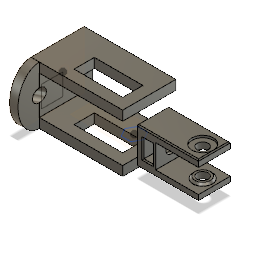
_Y Tensioner.c738b04c-2ad9-4713-af64-9a0c1ec9e032 (Autodesk Fusion 360 design; units mm, degrees)
Autodesk Fusion 360 part; units mm, degrees
sketch "Sketch1" plane through (0, 0, 0) normal (0, 0, 1) x (1, 0, 0)
  line L0 (0, 0) -> (29, 0)
  line L1 (29, 0) -> (29, 17)
  line L2 (29, 17) -> (0, 17)
  line L3 (0, 17) -> (0, 0)
  line L4 (8.977, 3) -> (29.9497, 3)
  line L5 (29.9497, 3) -> (29.9497, 14)
  line L6 (29.9497, 14) -> (8.977, 14)
  line L7 (8.977, 14) -> (8.977, 3)
  dimension "d1" = 17
  dimension "d2" = 29
  measures "d1" distance of L0.start
  measures "d2" distance of L0.start
extrude "Extrude1" add sketch "Sketch1" along normal blind 15 contours L0 L1 L2 L3 L4 L6 L7 makes body 1
sketch "Sketch2" plane through (0, 0, 0) normal (-1, 0, 0) x (0, 0, 1)
  line L0 (0, 17) -> (0, 0)
  line L1 (0, 0) -> (15, 0)
  line L2 (15, 0) -> (15, 17)
  line L3 (15, 17) -> (0, 17)
  circle A0 centre (7.5, 8.5) radius 3.1
  dimension "d5" = 6.2
  measures "d5" diameter of A0
extrude "Extrude2" cut sketch "Sketch2" against normal blind 3 draft -10 contours A0 bodies 1
sketch "Sketch3" plane through (0, 0, 0) normal (0, -1, 0) x (1, 0, 0)
  line L0 (0, 0) -> (29, 0)
  line L1 (29, 0) -> (29, 15)
  line L2 (29, 15) -> (0, 15)
  line L3 (0, 15) -> (0, 0)
  circle A0 centre (23.4671, 7.5) radius 2.6
  dimension "d8" = 5.2
  measures "d8" diameter of A0
extrude "Extrude3" cut sketch "Sketch3" against normal blind 17 contours A0 bodies 1
sketch "Sketch4" plane through (0, 14, 0) normal (0, -1, 0) x (1, 0, 0)
  circle A0 centre (23.4671, 7.5) radius 2.6
  line L0 (8.977, 0) -> (29, 0)
  line L1 (29, 0) -> (29, 15)
  line L2 (29, 15) -> (8.977, 15)
  line L3 (8.977, 15) -> (8.977, 0)
  circle A1 centre (23.4671, 7.5) radius 4.5
  dimension "d11" = 9
  measures "d11" diameter of A1
extrude "Extrude4" add sketch "Sketch4" along normal blind 1 contours A1 bodies 1
chamfer "Chamfer1" distance 0.9 angle 45 1 edges at (19.2716, 13, 5.8727) on bodies 1
sketch "Sketch5" plane through (0, 3, 0) normal (0, 1, 0) x (-1, 0, 0)
  circle A0 centre (-23.4671, 7.5) radius 2.6
  line L0 (-29, 0) -> (-8.977, 0)
  line L1 (-8.977, 0) -> (-8.977, 15)
  line L2 (-8.977, 15) -> (-29, 15)
  line L3 (-29, 15) -> (-29, 0)
  circle A1 centre (-23.4671, 7.5) radius 4.5
  dimension "d15" = 9
  measures "d15" diameter of A1
extrude "Extrude5" add sketch "Sketch5" along normal blind 1 contours A1 bodies 1
chamfer "Chamfer2" distance 0.9 angle 45 1 edges at (27.6626, 4, 5.8727) on bodies 1
sketch "Sketch6" plane through (8.977, 0, 0) normal (1, 0, 0) x (0, 0, -1)
  line L0 (0, 3) -> (0, 14)
  line L1 (0, 14) -> (-15, 14)
  line L2 (-15, 14) -> (-15, 3)
  line L3 (-15, 3) -> (0, 3)
  line L4 (-11.75, 4.25) -> (-3.25, 4.25)
  line L5 (-3.25, 12.75) -> (-11.75, 12.75)
  line L6 (-11.75, 4.25) -> (-3.25, 12.75) construction
  line L7 (-3.25, 4.25) -> (-11.75, 12.75) construction
  line L8 (-5.0463, 12.75) -> (-9.9537, 12.75)
  line L9 (-9.9537, 4.25) -> (-5.0463, 4.25)
  line L10 (-9.9537, 12.75) -> (-16, 12.75)
  line L11 (-16, 12.75) -> (-16, 4.25)
  line L12 (-16, 4.25) -> (-11.75, 4.25)
  line L13 (-2.5925, 8.5) -> (-3.25, 9.6388)
  line L14 (-3.25, 4.25) -> (-3.25, 7.3612)
  line L15 (-3.25, 9.6388) -> (-3.25, 12.75)
  line L16 (-3.25, 7.3612) -> (-2.5925, 8.5)
  dimension "d19" = 8.5
  dimension "d20" = 8.5
extrude "Extrude6" cut sketch "Sketch6" against normal blind 6 contours L2 L4 L5 L8 L9 L10 L12 L13 L14 L15 L16 bodies 1
sketch "Sketch13" plane through (8.977, 0, 0) normal (1, 0, 0) x (0, 0, -1)
  line L0 (-3.25, 4.25) -> (-15, 4.25)
  line L1 (-15, 4.25) -> (-15, 3)
  line L2 (-15, 3) -> (0, 3)
  line L3 (0, 3) -> (0, 14)
  line L4 (0, 14) -> (-15, 14)
  line L5 (-15, 14) -> (-15, 12.75)
  line L6 (-15, 12.75) -> (-3.25, 12.75)
  line L7 (-3.25, 12.75) -> (-3.25, 9.6388)
  line L8 (-3.25, 9.6388) -> (-2.5925, 8.5)
  line L9 (-2.5925, 8.5) -> (-3.25, 7.3612)
  line L10 (-3.25, 7.3612) -> (-3.25, 4.25)
  line L11 (0, 14) -> (-15, 14)
  line L12 (-15, 14) -> (-15, 3)
  line L13 (-15, 3) -> (0, 3)
  line L14 (0, 3) -> (0, 14)
extrude "Extrude13" add sketch "Sketch13" against normal blind 1.5 contours L0 L6 L7 L8 L9 L10 L12 bodies 1
chamfer "Chamfer6" distance 0.5 angle 45 14 edges at (14.5, 0, 15) (0, 0, 7.5) (14.5, 0, 0) (29, 0, 7.5) (0, 8.5, 15) (0, 8.5, 0) (0, 17, 7.5) (2.977, 8.5, 15) (5.227, 12.75, 15) (7.477, 8.5, 15) (5.227, 4.25, 15) (14.5, 17, 0) (29, 17, 7.5) (14.5, 17, 15) on bodies 1
sketch "Sketch14" plane through (8.977, 0, 0) normal (1, 0, 0) x (0, 0, -1)
  line L0 (-15, 14) -> (-15, 3)
  line L1 (-15, 3) -> (0, 3)
  line L2 (0, 3) -> (0, 14)
  line L3 (0, 14) -> (-15, 14)
  circle A0 centre (-7.5, 8.5775) radius 2.75
  dimension "d54" = 5.5
  measures "d54" diameter of A0
extrude "Extrude14" cut sketch "Sketch14" against normal blind 2 contours A0 bodies 1
sketch "Sketch15" plane through (0, 17, 0) normal (0, 1, 0) x (-1, 0, 0)
  circle A0 centre (-23.4671, 7.5) radius 2.6
  line L0 (-28.5, 0.5) -> (-0.5, 0.5)
  line L1 (-0.5, 0.5) -> (-0.5, 14.5)
  line L2 (-0.5, 14.5) -> (-28.5, 14.5)
  line L3 (-28.5, 14.5) -> (-28.5, 0.5)
  circle A1 centre (-23.4671, 7.5) radius 5
  dimension "d57" = 10
  measures "d57" diameter of A1
extrude "Extrude15" cut sketch "Sketch15" against normal blind 1 contours A1 bodies 1
sketch "Sketch16" plane through (0, 0, 0) normal (0, -1, 0) x (1, 0, 0)
  circle A0 centre (23.4671, 7.5) radius 2.6
  line L0 (0.5, 0.5) -> (28.5, 0.5)
  line L1 (28.5, 0.5) -> (28.5, 14.5)
  line L2 (28.5, 14.5) -> (0.5, 14.5)
  line L3 (0.5, 14.5) -> (0.5, 0.5)
  line L4 (18.9671, 7.5) -> (21.2171, 3.6029)
  line L5 (21.2171, 3.6029) -> (25.7171, 3.6029)
  line L6 (25.7171, 3.6029) -> (27.9671, 7.5)
  line L7 (27.9671, 7.5) -> (25.7171, 11.3971)
  line L8 (25.7171, 11.3971) -> (21.2171, 11.3971)
  line L9 (21.2171, 11.3971) -> (18.9671, 7.5)
  dimension "d63" = 4.5
extrude "Extrude17" cut sketch "Sketch16" against normal blind 1 contours L4 L5 L6 L7 L8 L9 bodies 1
extrude "Extrude16" cut sketch "Sketch16" against normal blind 1 contours L4 L5 L6 L7 L8 L9 bodies 1
sketch "Sketch7" plane through (0, 0, 0) normal (0, 0, 1) x (1, 0, 0)
  line L0 (33, 22) -> (-10, 22)
  line L1 (-10, 22) -> (-10, -5)
  line L2 (-10, -5) -> (33, -5)
  line L3 (33, -5) -> (33, 22)
  line L4 (-6.0376, -0.5) -> (33.9624, -0.5)
  line L5 (33.9624, -0.5) -> (33.9624, 17.5)
  line L6 (33.9624, 17.5) -> (-6.0376, 17.5)
  line L7 (-6.0376, 17.5) -> (-6.0376, -0.5)
  line L8 (-6.0376, -0.5) -> (33.9624, 17.5) construction
  line L9 (33.9624, -0.5) -> (-6.0376, 17.5) construction
  dimension "d23" = 18
  dimension "d24" = 40
  measures "d23" distance of origin
extrude "Extrude7" add sketch "Sketch7" along normal blind 25 separate body contours L0 L1 L2 L3 L4 L6 L7 makes body 2
move_body "Move1" bodies 2 to x (1, 0, 0) y (0, 1, 0) z (0, 0, 1) at (0, 0, -2.5)
sketch "Sketch8" plane through (-10, 0, 0) normal (-1, 0, 0) x (0, 0, 1)
  line L0 (-2.5, 22) -> (-2.5, -5)
  line L1 (-2.5, -5) -> (22.5, -5)
  line L2 (22.5, -5) -> (22.5, 22)
  line L3 (22.5, 22) -> (-2.5, 22)
  circle A0 centre (7.5, 8.4834) radius 2.65
  dimension "d27" = 5.3
  measures "d27" diameter of A0
extrude "Extrude8" cut sketch "Sketch8" against normal blind 4 contours A0 bodies 2
move_body "Move2" bodies 1 to x (1, 0, 0) y (0, 1, 0) z (0, 0, 1) at (0, 0, 5)
sketch "Sketch9" plane through (0, 22, 0) normal (0, 1, 0) x (-1, 0, 0)
  line L0 (-33, -2.5) -> (10, -2.5)
  line L1 (10, -2.5) -> (10, 22.5)
  line L2 (10, 22.5) -> (-33, 22.5)
  line L3 (-33, 22.5) -> (-33, -2.5)
  line L4 (-33, 22.5) -> (-22.9998, 12.5)
  line L5 (-18.2498, 17.25) -> (-27.7498, 17.25)
  line L6 (-27.7498, 17.25) -> (-27.7498, 7.75)
  line L7 (-27.7498, 7.75) -> (-18.2498, 7.75)
  line L8 (-18.2498, 7.75) -> (-18.2498, 17.25)
  line L9 (-18.2498, 17.25) -> (-27.7498, 7.75) construction
  line L10 (-27.7498, 17.25) -> (-18.2498, 7.75) construction
  line L11 (-18.2498, 7.75) -> (-5, 7.75)
  line L12 (-5, 7.75) -> (-5, 17.25)
  line L13 (-5, 17.25) -> (-18.2498, 17.25)
  dimension "d31" = 9.5
  dimension "d32" = 9.5
move_body "Move3" bodies 1 to x (1, 0, 0) y (0, 1, 0) z (0, 0, 1) at (37, 0, 0)
extrude "Extrude9" cut sketch "Sketch9" against normal blind 27 contours L5 L6 L7 L8 | L8 L11 L12 L13 bodies 2
sketch "Sketch10" plane through (-10, 0, 0) normal (-1, 0, 0) x (0, 0, 1)
  circle A0 centre (7.5, 8.4834) radius 2.65
  line L0 (-2.5, 22) -> (-2.5, -5)
  line L1 (-2.5, -5) -> (22.5, -5)
  line L2 (22.5, -5) -> (22.5, 22)
  line L3 (22.5, 22) -> (-2.5, 22)
  ellipse E0 centre (22.5, 8.5) end of major axis (22.5, -5) minor radius 10
  line L4 (22.5, 22) -> (22.5, -5)
  line L5 (12.5, 8.5) -> (32.5, 8.5)
  dimension "d35" = 20
extrude "Extrude10" add sketch "Sketch10" against normal blind 4 contours L2 E0 L4 L5 | L2 E0 L4 L5 picked at (29.1108, 9.3203) picked at (29.1307, 7.8405) bodies 2
sketch "Sketch17" plane through (-6, 0, 0) normal (1, 0, 0) x (0, 0, -1)
  ellipse E0 centre (-22.5, 8.5) end of major axis (-22.5, -5) minor radius 10 (-22.5, 22) -> (-22.5, -5) ccw
  line L0 (-22.5, -5) -> (-22.5, -0.5)
  line L1 (-22.5, -0.5) -> (-22.5, 17.5)
  line L2 (-22.5, 17.5) -> (-22.5, 22)
  circle A0 centre (-25.5, 8.5) radius 3
extrude "Extrude18" add sketch "Sketch17" along normal blind 5 and the other way blind 10 separate body contours A0 makes body 3
sketch "Sketch18" plane through (-10, 0, 0) normal (-1, 0, 0) x (0, 0, 1)
  circle A0 centre (7.5, 8.4834) radius 2.65
  line L0 (-2.5, 22) -> (-2.5, -5)
  line L1 (-2.5, -5) -> (22.5, -5)
  ellipse E0 centre (22.5, 8.5) end of major axis (22.5, -5) minor radius 10 (22.5, -5) -> (22.5, 22) ccw
  line L2 (22.5, 22) -> (-2.5, 22)
  line L3 (7.5, 8.4834) -> (17.5, 8.4834)
  line L4 (17.5, 8.4834) -> (17.5, -1.5166)
  line L5 (17.5, -1.5166) -> (7.5, -1.5166)
  line L6 (7.5, -1.5166) -> (7.5, 8.4834)
  dimension "d70" = 10
  dimension "d71" = 10
move_body "Move5" bodies 3 to x (0.906308, 0, -0.422618) y (0, 1, 0) z (0.422618, 0, 0.906308) at (-10.1431, 0, -3.768)
combine "Combine1" operation cut target body 2 tool bodies 3
extrude "Extrude12" [rolled back] along distance -5 taper angle 0
extrude "Extrude11" [rolled back] along distance -4.5 taper angle 0
chamfer "Chamfer3" [rolled back] left distance 2.5
chamfer "Chamfer4" [rolled back] left distance 2
fillet "Fillet1" [rolled back] radius 2
chamfer "Chamfer5" [rolled back] left distance 1
move_body "Move4" [rolled back]
sketch "Sketch12" plane through (0, 0, 0) normal (0, 1, 0) x (1, 0, 0)
equation "d51 = -6 mm + 4.5 mm"
equation "d63 = ( 9 / 2 ) * 1 mm"
named bodies: "tensioner", "mount"
